1.3mm_closerbottom (Autodesk Fusion 360 design; units mm, degrees)
Autodesk Fusion 360 part; units mm, degrees
sketch "Sketch1" plane through (0, 0, 0) normal (0, 1, 0) x (1, 0, 0)
  line L0 (0, 0) -> (0, -10)
  line L1 (0, -10) -> (-4, -10)
  line L2 (-4, -10) -> (-4, -7)
  line L3 (-4, -7) -> (-9, -7)
  line L4 (-9, -7) -> (-9, -0.9)
  line L5 (-9, -0.9) -> (-4, -0.9)
  line L6 (-4, -0.9) -> (-4, 0)
  line L7 (-4, 0) -> (0, 0)
  dimension "d1" = 4
  dimension "d2" = 10
  dimension "d3" = 7
  dimension "d4" = 4
  dimension "d5" = 5
  dimension "d6" = 0.9
  constraint coincident L0.start L7.end
  constraint vertical L0
  constraint perpendicular L0 L1
  constraint perpendicular L1 L2
  constraint perpendicular L2 L3
  constraint perpendicular L3 L4
  constraint perpendicular L4 L5
  constraint perpendicular L5 L6
  constraint perpendicular L0 L7
  measures "d1" distance of L6.end L0.start
  measures "d2" distance of L0.start L0.end
  measures "d3" distance of L0.start L3
  measures "d4" distance of L0.end L1.end
  measures "d5" distance of L2.end L3.end
  measures "d6" distance of L0.start L5
revolve "Revolve1" add sketch "Sketch1" angle 360 about axis through (1.75, 0, 0) along (1, 0, 0)
sketch "Sketch2" plane through (0, 0, 0) normal (1, 0, 0) x (0, 1, 0)
  line L0 (-5, -5.3364) -> (5.1728, -5.3364) construction
  line L1 (5.1728, -5.3364) -> (5.1728, 5) construction
  line L2 (5.1728, 5) -> (-5, 5) construction
  line L3 (-5, 5) -> (-5, -5.3364) construction
  circle A0 centre (0, 0) radius 10
  dimension "d10" = 3
  text T0 "1.3 mm" font "Arial" height 3 align centre middle in box 10.1728 x 10.3364 at (-5, -5.3364) x (1, 0) y (0, 1) spacing 1
emboss "Emboss1" depth 0.4 profiles "Sketch2" section 1 text T0 onto face at (0, 1.6236, 1.9302)
fillet "Fillet1" radius 0.5 4 edges at (-9, -2.5313, -6.5263) (-4, -2.5313, -6.5263) (-4, -3.6162, -9.3233) (0, -3.6162, -9.3233)
equation "d3 = ( 14 / 2 ) * 1 mm"
equation "d6 = 1.8 mm / 2"
